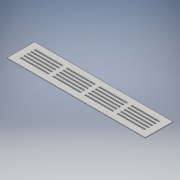
# Autodesk Inventor part: 28 inch grill
Saved by Autodesk Inventor 2017 (Build 210142000, 142)
## iProperties
Created: 2017-08-29
Part Number: 28 inch grill
Material: Generic
Document SubType Name: Modeling
Designer: mcgratta
Density: 1 g/cm^3
Appearance: Default
Author: mcgratta
Autodesk Inventor part; units mm, degrees
ref_plane "YZ Plane" through (0, 0, 0) normal (1, 0, 0) x (0, 1, 0)
ref_plane "XZ Plane" through (0, 0, 0) normal (0, 1, 0) x (-1, 0, 0)
ref_plane "XY Plane" through (0, 0, 0) normal (0, 0, 1) x (1, 0, 0)
sketch "Sketch1" plane through (0, 0, 0) normal (0, 1, 0) x (-1, 0, 0)
  line L0 (0, 0) -> (-762, 0)
  line L1 (-762, 0) -> (-762, -152.4)
  line L2 (-762, -152.4) -> (0, -152.4)
  line L3 (0, -152.4) -> (0, 0)
  line L4 (-25.4, -25.4) -> (-736.6, -25.4)
  line L5 (-736.6, -25.4) -> (-736.6, -127)
  line L6 (-736.6, -127) -> (-25.4, -127)
  line L7 (-25.4, -127) -> (-25.4, -25.4)
  line L8 (-38.1, -117.475) -> (-190.5, -117.475)
  line L9 (-190.5, -117.475) -> (-190.5, -111.125)
  line L10 (-190.5, -111.125) -> (-38.1, -111.125)
  line L11 (-38.1, -111.125) -> (-38.1, -117.475)
  line L12 (-38.1, -98.425) -> (-190.5, -98.425)
  line L13 (-190.5, -98.425) -> (-190.5, -92.075)
  line L14 (-190.5, -92.075) -> (-38.1, -92.075)
  line L15 (-38.1, -92.075) -> (-38.1, -98.425)
  line L16 (-38.1, -79.375) -> (-190.5, -79.375)
  line L17 (-190.5, -79.375) -> (-190.5, -73.025)
  line L18 (-190.5, -73.025) -> (-38.1, -73.025)
  line L19 (-38.1, -73.025) -> (-38.1, -79.375)
  line L20 (-38.1, -60.325) -> (-190.5, -60.325)
  line L21 (-190.5, -60.325) -> (-190.5, -53.975)
  line L22 (-190.5, -53.975) -> (-38.1, -53.975)
  line L23 (-38.1, -53.975) -> (-38.1, -60.325)
  line L24 (-38.1, -41.275) -> (-190.5, -41.275)
  line L25 (-190.5, -41.275) -> (-190.5, -34.925)
  line L26 (-190.5, -34.925) -> (-38.1, -34.925)
  line L27 (-38.1, -34.925) -> (-38.1, -41.275)
  line L28 (-215.9, -117.475) -> (-368.3, -117.475)
  line L29 (-368.3, -117.475) -> (-368.3, -111.125)
  line L30 (-368.3, -111.125) -> (-215.9, -111.125)
  line L31 (-215.9, -111.125) -> (-215.9, -117.475)
  line L32 (-215.9, -92.075) -> (-215.9, -98.425)
  line L33 (-215.9, -98.425) -> (-368.3, -98.425)
  line L34 (-368.3, -98.425) -> (-368.3, -92.075)
  line L35 (-368.3, -92.075) -> (-215.9, -92.075)
  line L36 (-215.9, -73.025) -> (-215.9, -79.375)
  line L37 (-215.9, -79.375) -> (-368.3, -79.375)
  line L38 (-368.3, -79.375) -> (-368.3, -73.025)
  line L39 (-368.3, -73.025) -> (-215.9, -73.025)
  line L40 (-215.9, -53.975) -> (-215.9, -60.325)
  line L41 (-215.9, -60.325) -> (-368.3, -60.325)
  line L42 (-368.3, -60.325) -> (-368.3, -53.975)
  line L43 (-368.3, -53.975) -> (-215.9, -53.975)
  line L44 (-215.9, -34.925) -> (-215.9, -41.275)
  line L45 (-215.9, -41.275) -> (-368.3, -41.275)
  line L46 (-368.3, -41.275) -> (-368.3, -34.925)
  line L47 (-368.3, -34.925) -> (-215.9, -34.925)
  line L48 (-393.7, -117.475) -> (-546.1, -117.475)
  line L49 (-546.1, -117.475) -> (-546.1, -111.125)
  line L50 (-546.1, -111.125) -> (-393.7, -111.125)
  line L51 (-393.7, -111.125) -> (-393.7, -117.475)
  line L52 (-393.7, -92.075) -> (-393.7, -98.425)
  line L53 (-393.7, -98.425) -> (-546.1, -98.425)
  line L54 (-546.1, -98.425) -> (-546.1, -92.075)
  line L55 (-546.1, -92.075) -> (-393.7, -92.075)
  line L56 (-393.7, -73.025) -> (-393.7, -79.375)
  line L57 (-393.7, -79.375) -> (-546.1, -79.375)
  line L58 (-546.1, -79.375) -> (-546.1, -73.025)
  line L59 (-546.1, -73.025) -> (-393.7, -73.025)
  line L60 (-393.7, -53.975) -> (-393.7, -60.325)
  line L61 (-393.7, -60.325) -> (-546.1, -60.325)
  line L62 (-546.1, -60.325) -> (-546.1, -53.975)
  line L63 (-546.1, -53.975) -> (-393.7, -53.975)
  line L64 (-393.7, -34.925) -> (-393.7, -41.275)
  line L65 (-393.7, -41.275) -> (-546.1, -41.275)
  line L66 (-546.1, -41.275) -> (-546.1, -34.925)
  line L67 (-546.1, -34.925) -> (-393.7, -34.925)
  line L68 (-571.5, -117.475) -> (-723.9, -117.475)
  line L69 (-723.9, -117.475) -> (-723.9, -111.125)
  line L70 (-723.9, -111.125) -> (-571.5, -111.125)
  line L71 (-571.5, -111.125) -> (-571.5, -117.475)
  line L72 (-571.5, -92.075) -> (-571.5, -98.425)
  line L73 (-571.5, -98.425) -> (-723.9, -98.425)
  line L74 (-723.9, -98.425) -> (-723.9, -92.075)
  line L75 (-723.9, -92.075) -> (-571.5, -92.075)
  line L76 (-571.5, -73.025) -> (-571.5, -79.375)
  line L77 (-571.5, -79.375) -> (-723.9, -79.375)
  line L78 (-723.9, -79.375) -> (-723.9, -73.025)
  line L79 (-723.9, -73.025) -> (-571.5, -73.025)
  line L80 (-571.5, -53.975) -> (-571.5, -60.325)
  line L81 (-571.5, -60.325) -> (-723.9, -60.325)
  line L82 (-723.9, -60.325) -> (-723.9, -53.975)
  line L83 (-723.9, -53.975) -> (-571.5, -53.975)
  line L84 (-571.5, -34.925) -> (-571.5, -41.275)
  line L85 (-571.5, -41.275) -> (-723.9, -41.275)
  line L86 (-723.9, -41.275) -> (-723.9, -34.925)
  line L87 (-723.9, -34.925) -> (-571.5, -34.925)
  dimension "d0" = 762
  dimension "d1" = 152.4
  dimension "d2" = 25.4
  dimension "d3" = 25.4
  dimension "d4" = 25.4
  dimension "d5" = 25.4
  dimension "d6" = 6.35
  dimension "d7" = 12.7
  dimension "d8" = 9.525
  dimension "d9" = 152.4
  dimension "d10" = 6.35
  dimension "d11" = 152.4
  dimension "d12" = 6.35
  dimension "d13" = 152.4
  dimension "d14" = 6.35
  dimension "d15" = 152.4
  dimension "d16" = 6.35
  dimension "d17" = 152.4
  dimension "d18" = 12.7
  dimension "d19" = 12.7
  dimension "d20" = 12.7
  dimension "d21" = 12.7
  dimension "d22" = 12.7
  dimension "d23" = 12.7
  dimension "d24" = 12.7
  dimension "d25" = 12.7
  dimension "d26" = 6.35
  dimension "d27" = 152.4
  dimension "d28" = 6.35
  dimension "d29" = 152.4
  dimension "d30" = 6.35
  dimension "d31" = 152.4
  dimension "d32" = 6.35
  dimension "d33" = 152.4
  dimension "d34" = 6.35
  dimension "d35" = 152.4
  dimension "d36" = 12.7
  dimension "d37" = 12.7
  dimension "d38" = 12.7
  dimension "d39" = 12.7
  dimension "d40" = 6.35
  dimension "d41" = 152.4
  dimension "d42" = 6.35
  dimension "d43" = 152.4
  dimension "d44" = 6.35
  dimension "d45" = 152.4
  dimension "d46" = 6.35
  dimension "d47" = 152.4
  dimension "d48" = 6.35
  dimension "d49" = 152.4
  dimension "d50" = 12.7
  dimension "d51" = 12.7
  dimension "d52" = 12.7
  dimension "d53" = 12.7
  dimension "d54" = 6.35
  dimension "d55" = 152.4
  dimension "d56" = 6.35
  dimension "d57" = 152.4
  dimension "d58" = 6.35
  dimension "d59" = 152.4
  dimension "d60" = 6.35
  dimension "d61" = 152.4
  dimension "d62" = 6.35
  dimension "d63" = 152.4
  constraints: 176 end point, 44 parallel, 22 horizontal, 22 perpendicular
  measures "d0" distance of L1.end L2.end
  measures "d1" distance of L0.end L1.end
  measures "d2" distance between parallel lines of L3 L7
  measures "d3" distance between parallel lines of L6 L2
  measures "d4" distance between parallel lines of L0 L4
  measures "d5" distance between parallel lines of L1 L5
  measures "d6" distance between parallel lines of L10 L8
  measures "d7" distance between parallel lines of L11 L7
  measures "d8" distance between parallel lines of L8 L6
  measures "d9" distance between parallel lines of L9 L11
  measures "d10" distance between parallel lines of L14 L12
  measures "d11" distance between parallel lines of L13 L15
  measures "d12" distance between parallel lines of L18 L16
  measures "d13" distance between parallel lines of L17 L19
  measures "d14" distance between parallel lines of L22 L20
  measures "d15" distance between parallel lines of L21 L23
  measures "d16" distance between parallel lines of L26 L24
  measures "d17" distance between parallel lines of L25 L27
  measures "d18" distance between parallel lines of L12 L10
  measures "d19" distance between parallel lines of L16 L14
  measures "d20" distance between parallel lines of L20 L18
  measures "d21" distance between parallel lines of L24 L22
  measures "d22" distance between parallel lines of L15 L7
  measures "d23" distance between parallel lines of L19 L7
  measures "d24" distance between parallel lines of L7 L23
  measures "d25" distance between parallel lines of L7 L27
  measures "d26" distance between parallel lines of L30 L28
  measures "d27" distance between parallel lines of L29 L31
  measures "d28" distance between parallel lines of L35 L33
  measures "d29" distance between parallel lines of L34 L32
  measures "d30" distance between parallel lines of L39 L37
  measures "d31" distance between parallel lines of L38 L36
  measures "d32" distance between parallel lines of L43 L41
  measures "d33" distance between parallel lines of L42 L40
  measures "d34" distance between parallel lines of L47 L45
  measures "d35" distance between parallel lines of L46 L44
  measures "d36" distance between parallel lines of L33 L30
  measures "d37" distance between parallel lines of L37 L35
  measures "d38" distance between parallel lines of L41 L39
  measures "d39" distance between parallel lines of L45 L43
  measures "d40" distance between parallel lines of L50 L48
  measures "d41" distance between parallel lines of L49 L51
  measures "d42" distance between parallel lines of L55 L53
  measures "d43" distance between parallel lines of L54 L52
  measures "d44" distance between parallel lines of L59 L57
  measures "d45" distance between parallel lines of L58 L56
  measures "d46" distance between parallel lines of L63 L61
  measures "d47" distance between parallel lines of L62 L60
  measures "d48" distance between parallel lines of L67 L65
  measures "d49" distance between parallel lines of L66 L64
  measures "d50" distance between parallel lines of L53 L50
  measures "d51" distance between parallel lines of L57 L55
  measures "d52" distance between parallel lines of L61 L59
  measures "d53" distance between parallel lines of L65 L63
  measures "d54" distance between parallel lines of L70 L68
  measures "d55" distance between parallel lines of L69 L71
  measures "d56" distance between parallel lines of L75 L73
  measures "d57" distance between parallel lines of L74 L72
  measures "d58" distance between parallel lines of L79 L77
  measures "d59" distance between parallel lines of L78 L76
  measures "d60" distance between parallel lines of L83 L81
  measures "d61" distance between parallel lines of L82 L80
  measures "d62" distance between parallel lines of L87 L85
  measures "d63" distance between parallel lines of L86 L84
extrude "Extrusion1" add sketch "Sketch1" along normal blind 3.175 contours L3 L2 L1 L0 | L7 L6 L5 L4
body "Solid1"
